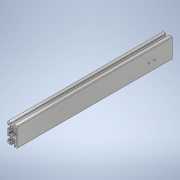
# Autodesk Inventor part: HFSF5-2040-320-TPW
Saved by Autodesk Inventor 2022 (Build 260153000, 153)
## iProperties
Category: PARTsolutions
Company: MISUMI
Created: 2022-12-05
Part Number: HFSF5-2040-320-TPW
Material: Generic
Catalog Web Link: www.cadenas.de
Description: NFS5-2040, NFSB5-2040, HFS5-2040, HFSB5-2040, CAF5-2040, NFSF5-2040, HFSF5-2040, HFSY5-2040-Aluminum Frames -5 Series-2Row Groove 20x40 mm Square -Specified Length
Vendor: MISUMI
Document SubType Name: Modeling
Designer: psAdmin
Manufacturer: MISUMI
Mass: 109.926 g
Surface Area: 1036.55 cm^2
Volume: 109.926 cm^3
Density: 1 g/cm^3
Appearance: アルミニウム - つや出し
PSOL_IDENT_0: {$CADENAS_DATA/23d-libs/misumi/metric/38_al_extrusions_blackets/5/hfs5_2040.prj},636 {VTYP=3D},{NB=H
PSOL_IDENT_1: FSF5-2040-320-TPW},{LINA=HFSF5-2040-320-TPW},{NN=NFS5-2040, NFSB5-2040, HFS5-2040, HFSB5-2040, CAF5-
PSOL_IDENT_2: 2040, NFSF5-2040, HFSF5-2040, HFSY5-2040},{DATE=30.11.2021 06:05:55},{GEOMDATE=23.09.2021 02:57:03},
PSOL_IDENT_3: {VERSION=},{LINEID=30},{WBVAR=L,ALT1,ALT2,ALT4,ALT5,CP5,DL5,DR5,ALT6,ALT9,ALT10,ALT11,HP6,NHL6,DL6,N
PSOL_IDENT_4: HR6,DR6,ALT7,ALT8,NH9,AH,BH,CH,DH,EH,NH10,AV,BV,CV,DV,EV,NH11,AP,BP,CP,DP,EP,ALT12,ALT13,Z,NH12,XA,X
PSOL_IDENT_5: B,XC,XD,XE,NH13,YA,YB,YC,YD,YE,ALT16,HP16,DL16,DR16,ALT17,HQ17,JLP,ALT18,HQ18,KLP,ALT20},{WBNUMERIC=
PSOL_IDENT_6: L,NH9,AH,BH,CH,DH,EH,NH10,AV,BV,CV,DV,EV,NH11,AP,BP,CP,DP,EP,NH12,XA,XB,XC,XD,XE,NH13,YA,YB,YC,YD,YE
PSOL_IDENT_7: ,HQ17,JLP,HQ18,KLP}  {NB=HFSF5-2040-320-TPW},{LINA=HFSF5-2040-320-TPW},{KT=DUMMY},{PN=HFSF5-2040-320
PSOL_IDENT_8: -TPW},{TPS=HFSF5-2040},{MAT=A6N01SS-T5 Aluminum Alloy},{ST=Clear Anodize},{FRMW=20},{FRMH=40},{FRD=4
PSOL_IDENT_9: .2},{L=320},{MASS=0.93},{SA=344},{LX=1.52x10^4},{LY=5.40x10^4},{ALT1=TPW},{M1=5},{DPL1=15},{DPR1=15}
PSOL_IDENT_10: ,{ALT1PN=-TPW},{ALT2=},{ALT2ALG= '','Not applicable' },{M2=0},{DP2=0},{ALT2PN=},{ALT4=},{ALT4ALG= ''
PSOL_IDENT_11: , 'w/o SC (High Precision Cut)', 'SC', 'with SC (High Precision Cut)' },{ALT4PN=},{ALT5=},{ALT5ALG= ''
PSOL_IDENT_12: ,'w/o 45 Degree Cut','1','with 45 Degree Cut' },{CP5=},{CP5ALG= '','N/A' },{DL5=},{DL5ALG= '','N/A'
PSOL_IDENT_13: },{DR5=},{DR5ALG= '','N/A' },{FRMLALT5=0},{FRMRALT5=0},{ALT5PN=},{ALT6=},{ALT6ALG= '','w/o Fastening
PSOL_IDENT_14: Location Wrench Access Hole Alterations','1','with Fastening Location Wrench Access Hole Alteration
PSOL_IDENT_15: s' },{ALT9=},{ALT9ALG= '','w/o Location Specified Wrench Access Hole Alteratons (Horizontal)','1','w
PSOL_IDENT_16: ith Location Specified Wrench Access Hole Alteratons (Horizontal)' },{ALT10=},{ALT10ALG= '','w/o Loc
PSOL_IDENT_17: ation Specified Wrench Access Hole Alteratons (Vertical)','1','with Location Specified Wrench Access
PSOL_IDENT_18: Hole Alteratons (Vertical)' },{ALT11=},{ALT11ALG= '','w/o Location Specified Wrench Access Hole Alt
PSOL_IDENT_19: eratons (Crisscross)','1','with Location Specified Wrench Access Hole Alteratons (Crisscross)' },{HP
PSOL_IDENT_20: 6=},{HP6ALG= '','N/A' },{NHL6=},{NHL6ALG= '','N/A' },{DL6=},{DL6ALG= '','N/A' },{NHR6=},{NHR6ALG= ''
PSOL_IDENT_21: ,'N/A' },{DR6=},{DR6ALG= '','N/A' },{HL6=0},{HL6D=0},{HR6=0},{HR6D=0},{J6=0},{J6D=0},{K6=0},{K6D=0},
PSOL_IDENT_22: {DD6=0.00},{DD6ALG=0},{ALT7=},{ALT7ALG= '','N/A' },{ALT8=},{ALT8ALG= '','N/A' },{ALT678PN=},{NH9=0},
PSOL_IDENT_23: {NH9MAX=5},{NH9ALG=[0]},{AH=0.0},{AHMIN=7},{AHMAX=315},{AHALG=[0]},{BH=0.0},{BHMIN=2},{BHMAX=317},{B
PSOL_IDENT_24: HALG=[0]},{CH=0.0},{CHMIN=2},{CHMAX=319},{CHALG=[0]},{DH=0.0},{DHMIN=2},{DHMAX=321},{DHALG=[0]},{EH=
PSOL_IDENT_25: 0.0},{EHMIN=2},{EHMAX=313},{EHALG=[0]},{NH10=0},{NH10MAX=5},{NH10ALG=[0]},{AV=0.0},{AVMIN=7},{AVMAX=
PSOL_IDENT_26: 315},{AVALG=[0]},{BV=0.0},{BVMIN=2},{BVMAX=317},{BVALG=[0]},{CV=0.0},{CVMIN=2},{CVMAX=319},{CVALG=[0
PSOL_IDENT_27: ]},{DV=0.0},{DVMIN=2},{DVMAX=321},{DVALG=[0]},{EV=0.0},{EVMIN=2},{EVMAX=313},{EVALG=[0]},{NH11=0},{N
PSOL_IDENT_28: H11MAX=5},{NH11ALG=[0]},{AP=0.0},{APMIN=7},{APMAX=315},{APALG=[0]},{BP=0.0},{BPMIN=2},{BPMAX=317},{B
PSOL_IDENT_29: PALG=[0]},{CP=0.0},{CPMIN=2},{CPMAX=319},{CPALG=[0]},{DP=0.0},{DPMIN=2},{DPMAX=321},{DPALG=[0]},{EP=
PSOL_IDENT_30: 0.0},{EPMIN=2},{EPMAX=313},{EPALG=[0]},{ALT9PN=},{ALT10PN=},{ALT11PN=},{ALT91011PN=},{ALT12=},{ALT12
PSOL_IDENT_31: ALG= '','w/o Counterbore Hole in Specified Position (Vertical)','1','with Counterbore Hole in Specif
PSOL_IDENT_32: ied Position (Vertical)' },{ALT13=},{ALT13ALG= '','N/A' },{Z=},{ZALG= '','N/A' },{DD12=0.0},{DD112=0
PSOL_IDENT_33: .0},{NH12=0},{NH12MAX=5},{NH12ALG=[0]},{XA=0.0},{XAMIN=7},{XAMAX=315},{XAALG=[0]},{XB=0.0},{XBMIN=2}
PSOL_IDENT_34: ,{XBMAX=317},{XBALG=[0]},{XC=0.0},{XCMIN=2},{XCMAX=319},{XCALG=[0]},{XD=0.0},{XDMIN=2},{XDMAX=321},{
PSOL_IDENT_35: XDALG=[0]},{XE=0.0},{XEMIN=2},{XEMAX=313},{XEALG=[0]},{NH13=0},{NH13MAX=5},{NH13ALG=[0]},{YA=0.0},{Y
PSOL_IDENT_36: AMIN=7},{YAMAX=315},{YAALG=[0]},{YB=0.0},{YBMIN=2},{YBMAX=317},{YBALG=[0]},{YC=0.0},{YCMIN=2},{YCMAX=
PSOL_IDENT_37: 319},{YCALG=[0]},{YD=0.0},{YDMIN=2},{YDMAX=321},{YDALG=[0]},{YE=0.0},{YEMIN=2},{YEMAX=313},{YEALG=[0
PSOL_IDENT_38: ]},{ALT12PN=},{ALT13PN=},{ALT1213PN=},{ALT16=},{ALT16ALG= '','w/o M Type Hole Alteration','1','with
PSOL_IDENT_39: M Type Hole Alteration' },{HP16=},{HP16ALG= '','N/A' },{DL16=},{DL16ALG= '','N/A' },{DR16=},{DR16ALG=
PSOL_IDENT_40: '','N/A' },{H116=0},{D16=0.0},{ALT16PN=},{ALT17=},{ALT17ALG= '','w/o L Type Hole Alteration (Top)','
PSOL_IDENT_41: 1','with L Type Hole Alteration (Top)' },{HQ17=0},{HQ17ALG=0},{JLP=0},{JLPMIN=4.9},{JLPMAX=0},{JLPAL
PSOL_IDENT_42: G=[0]},{L17=0},{D17=0.0},{ALT18=},{ALT18ALG= '','w/o L Type Hole Alteration (Bottom)','1','with L Ty
PSOL_IDENT_43: pe Hole Alteration (Bottom)' },{HQ18=0},{HQ18ALG=0},{KLP=0},{KLPMIN=4.9},{KLPMAX=0},{KLPALG=[0]},{L1
PSOL_IDENT_44: 8=0},{D18=0.0},{ALT1718PN=},{ALT20=},{ALT20PN=},{ERRORALT01=OK},{ERRORALT02=OK},{ERRORALT05=OK},{ERR
PSOL_IDENT_45: ORALT06091=OK},{ERRORALT06092=OK},{ERRORALT06093=OK},{ERRORALT06094=OK},{ERRORALT06101=OK},{ERRORALT
PSOL_IDENT_46: 06102=OK},{ERRORALT06103=OK},{ERRORALT06104=OK},{ERRORALT06111=OK},{ERRORALT06112=OK},{ERRORALT06113=
PSOL_IDENT_47: OK},{ERRORALT06114=OK},{ERRORALT06121=OK},{ERRORALT06122=OK},{ERRORALT06123=OK},{ERRORALT06124=OK},{
PSOL_IDENT_48: ERRORALT06131=OK},{ERRORALT06132=OK},{ERRORALT06133=OK},{ERRORALT06134=OK},{ERRORALT0616=OK},{ERRORA
PSOL_IDENT_49: LT06171=OK},{ERRORALT06172=OK},{ERRORALT06173=OK},{ERRORALT06181=OK},{ERRORALT06182=OK},{ERRORALT061
PSOL_IDENT_50: 83=OK},{ERRORALT0911=OK},{ERRORALT0913=OK},{ERRORALT0916=OK},{ERRORALT0917=OK},{ERRORALT0918=OK},{ER
PSOL_IDENT_51: RORALT1011=OK},{ERRORALT1012=OK},{ERRORALT1016=OK},{ERRORALT1017=OK},{ERRORALT1018=OK},{ERRORALT1112=
PSOL_IDENT_52: OK},{ERRORALT1113=OK},{ERRORALT1116=OK},{ERRORALT1117=OK},{ERRORALT1118=OK},{ERRORALT1216=OK},{ERROR
PSOL_IDENT_53: ALT1217=OK},{ERRORALT1218=OK},{ERRORALT1316=OK},{ERRORALT1317=OK},{ERRORALT1318=OK},{ERRORALT1617=OK
PSOL_IDENT_54: },{ERRORALT1618=OK},{ERRORPN=},{TFW=2},{COLOR=}
NB: HFSF5-2040-320-TPW
NN: NFS5-2040, NFSB5-2040, HFS5-2040, HFSB5-2040, CAF5-2040, NFSF5-2040, HFSF5-2040, HFSY5-2040
NT: Aluminum Frames -5 Series-2Row Groove 20x40 mm Square -Specified Length
NBSYN: $PN.
LINA: HFSF5-2040-320-TPW
CATALOG: Misumi
PN: HFSF5-2040-320-TPW
TPS: HFSF5-2040
MAT: A6N01SS-T5 Aluminum Alloy
ST: Clear Anodize
L: 320
MASS: 0.93
SA: 344
LX: 1.52x10^4
LY: 5.40x10^4
ALT1: with TPW (Tapping on Both Ends)
M1: 5
DPL1: 15
DPR1: 15
ALT2: Not applicable
M2: 0
DP2: 0
ALT4: w/o SC (High Precision Cut)
ALT5: w/o 45 Degree Cut
CP5: N/A
DL5: N/A
DR5: N/A
ALT6: w/o Fastening Location Wrench Access Hole Alterations
ALT9: w/o Location Specified Wrench Access Hole Alteratons (Horizontal)
ALT10: w/o Location Specified Wrench Access Hole Alteratons (Vertical)
ALT11: w/o Location Specified Wrench Access Hole Alteratons (Crisscross)
HP6: N/A
NHL6: N/A
DL6: N/A
NHR6: N/A
DR6: N/A
HL6D: 0
HR6D: 0
J6D: 0
K6D: 0
DD6: 0
ALT7: N/A
ALT8: N/A
NH9: 0
AH: 0
BH: 0
CH: 0
DH: 0
EH: 0
NH10: 0
AV: 0
BV: 0
CV: 0
DV: 0
EV: 0
NH11: 0
AP: 0
BP: 0
CP: 0
DP: 0
EP: 0
ALT12: w/o Counterbore Hole in Specified Position (Vertical)
ALT13: N/A
Z: N/A
DD12: 0
DD112: 0
NH12: 0
XA: 0
XB: 0
XC: 0
XD: 0
XE: 0
NH13: 0
YA: 0
YB: 0
YC: 0
YD: 0
YE: 0
ALT16: w/o M Type Hole Alteration
HP16: N/A
DL16: N/A
DR16: N/A
H116: 0
D16: 0
ALT17: w/o L Type Hole Alteration (Top)
HQ17: 0
JLP: 0
D17: 0
ALT18: w/o L Type Hole Alteration (Bottom)
HQ18: 0
KLP: 0
D18: 0
ALT20: w/o CW (End Face C Chamfering)
SUPPLIER: MISUMI
ARTICLENO: HFSF5-2040-320-TPW
BOMINFO: HFSF5-2040-320-TPW
CREATOR: CADENAS GmbH
Title: HFSF5-2040-320-TPW
Author: Cadenas PARTsolutions
Comments: Aluminum Frames -5 Series-2Row Groove 20x40 mm Square -Specified Length
Autodesk Inventor part; units mm, degrees
ref_plane "YZ Plane" through (0, 0, 0) normal (1, 0, 0) x (0, 1, 0)
ref_plane "XZ Plane" through (0, 0, 0) normal (0, 1, 0) x (-1, 0, 0)
ref_plane "XY Plane" through (0, 0, 0) normal (0, 0, 1) x (1, 0, 0)
sketch "Sketch_63" plane through (0, 0, 0) normal (0, 0, 1) x (1, 0, 0)
  line L0 (-10, -7) -> (-8, -7)
  line L1 (-8, -7) -> (-8, -4)
  line L2 (-8, -4) -> (-7.0607, -4)
  line L3 (-7.0607, -4) -> (-4, -7.0607)
  line L4 (-4, -7.0607) -> (-4, -9.4804)
  line L5 (-4, -9.4804) -> (-3.7, -10)
  line L6 (-3.7, -10) -> (-4, -10.5196)
  line L7 (-4, -10.5196) -> (-4, -12.9393)
  line L8 (-4, -12.9393) -> (-7.0607, -16)
  line L9 (-7.0607, -16) -> (-8, -16)
  line L10 (-8, -16) -> (-8, -13)
  line L11 (-8, -13) -> (-10, -13)
  line L12 (-10, -13) -> (-10, -19)
  arc A0 (-10, -19) -> (-9, -20) centre (-9, -19) ccw
  line L13 (-9, -20) -> (-3, -20)
  line L14 (-3, -20) -> (-3, -18)
  line L15 (-3, -18) -> (-6, -18)
  line L16 (-6, -18) -> (-6, -17.0607)
  line L17 (-6, -17.0607) -> (-2.9393, -14)
  line L18 (-2.9393, -14) -> (-0.5196, -14)
  line L19 (-0.5196, -14) -> (0, -13.7)
  line L20 (0, -13.7) -> (0.5196, -14)
  line L21 (0.5196, -14) -> (2.9393, -14)
  line L22 (2.9393, -14) -> (6, -17.0607)
  line L23 (6, -17.0607) -> (6, -18)
  line L24 (6, -18) -> (3, -18)
  line L25 (3, -18) -> (3, -20)
  line L26 (3, -20) -> (9, -20)
  arc A1 (9, -20) -> (10, -19) centre (9, -19) ccw
  line L27 (10, -19) -> (10, 19)
  arc A2 (10, 19) -> (9, 20) centre (9, 19) ccw
  line L28 (9, 20) -> (3, 20)
  line L29 (3, 20) -> (3, 18)
  line L30 (3, 18) -> (6, 18)
  line L31 (6, 18) -> (6, 17.0607)
  line L32 (6, 17.0607) -> (2.9393, 14)
  line L33 (2.9393, 14) -> (0.5196, 14)
  line L34 (0.5196, 14) -> (0, 13.7)
  line L35 (0, 13.7) -> (-0.5196, 14)
  line L36 (-0.5196, 14) -> (-2.9393, 14)
  line L37 (-2.9393, 14) -> (-6, 17.0607)
  line L38 (-6, 17.0607) -> (-6, 18)
  line L39 (-6, 18) -> (-3, 18)
  line L40 (-3, 18) -> (-3, 20)
  line L41 (-3, 20) -> (-9, 20)
  arc A3 (-9, 20) -> (-10, 19) centre (-9, 19) ccw
  line L42 (-10, 19) -> (-10, 13)
  line L43 (-10, 13) -> (-8, 13)
  line L44 (-8, 13) -> (-8, 16)
  line L45 (-8, 16) -> (-7.0607, 16)
  line L46 (-7.0607, 16) -> (-4, 12.9393)
  line L47 (-4, 12.9393) -> (-4, 10.5196)
  line L48 (-4, 10.5196) -> (-3.7, 10)
  line L49 (-3.7, 10) -> (-4, 9.4804)
  line L50 (-4, 9.4804) -> (-4, 7.0607)
  line L51 (-4, 7.0607) -> (-7.0607, 4)
  line L52 (-7.0607, 4) -> (-8, 4)
  line L53 (-8, 4) -> (-8, 7)
  line L54 (-8, 7) -> (-10, 7)
  line L55 (-10, 7) -> (-10, -7)
  line L56 (4, 12.9393) -> (4, 8.5)
  arc A4 (4, 8.5) -> (5, 7.5) centre (5, 8.5) ccw
  line L57 (5, 7.5) -> (7, 7.5)
  arc A5 (7, 7.5) -> (8, 8.5) centre (7, 8.5) ccw
  line L58 (8, 8.5) -> (8, 16)
  line L59 (8, 16) -> (7.0607, 16)
  line L60 (7.0607, 16) -> (4, 12.9393)
  line L61 (4, -12.9393) -> (7.0607, -16)
  line L62 (7.0607, -16) -> (8, -16)
  line L63 (8, -16) -> (8, -8.5)
  arc A6 (8, -8.5) -> (7, -7.5) centre (7, -8.5) ccw
  line L64 (7, -7.5) -> (5, -7.5)
  arc A7 (5, -7.5) -> (4, -8.5) centre (5, -8.5) ccw
  line L65 (4, -8.5) -> (4, -12.9393)
  line L66 (-8, 1.7) -> (-8, -1.7)
  arc A8 (-8, -1.7) -> (-7.7, -2) centre (-7.7, -1.7) ccw
  line L67 (-7.7, -2) -> (-7.0636, -2)
  arc A9 (-6.8515, -2.0879) -> (-7.0636, -2) centre (-7.0636, -2.3) ccw
  line L68 (-6.8515, -2.0879) -> (-2.9393, -6)
  line L69 (-2.9393, -6) -> (7, -6)
  arc A10 (7, -6) -> (8, -5) centre (7, -5) ccw
  line L70 (8, -5) -> (8, 5)
  arc A11 (8, 5) -> (7, 6) centre (7, 5) ccw
  line L71 (7, 6) -> (-2.9393, 6)
  line L72 (-2.9393, 6) -> (-6.8515, 2.0879)
  arc A12 (-7.0636, 2) -> (-6.8515, 2.0879) centre (-7.0636, 2.3) ccw
  line L73 (-7.0636, 2) -> (-7.7, 2)
  arc A13 (-7.7, 2) -> (-8, 1.7) centre (-7.7, 1.7) ccw
  constraints: 148 end point, 28 point on circle, 14 centre point
extrude "Extrusion1" add sketch "Sketch_63" against normal blind 320
sketch "Sketch2" plane through (0, 0, 0) normal (0, 0, 1) x (1, 0, 0)
  point P0 (0, 10)
hole "Hole1" at (0, 10, 0) direction (0, 0, -1) diameter 4.134 depth 15 countersink diameter 5 countersink angle 90 thread size "M5x0.8" class "6H" standard "ISO Metric profile"
pattern_linear "Rectangular Pattern1" count 2 spacing 20 along (0, -1, 0) of "Hole1"
sketch "Sketch3" plane through (0, 0, -320) normal (0, 0, -1) x (-1, 0, 0)
  point P0 (0, 10)
hole "Hole2" at (0, 10, -320) direction (0, 0, 1) diameter 4.134 depth 15 countersink diameter 5 countersink angle 90 thread size "M5x0.8" class "6H" standard "ISO Metric profile"
pattern_linear "Rectangular Pattern2" count 2 spacing 20 along (0, -1, 0) of "Hole2"
sketch "Sketch4" plane through (0, 10, -305) normal (0, 0, -1) x (-1, 0, 0)
  point P0 (0, 0)
hole "Hole3" at (0, 10, -305) direction (0, 0, 1) diameter 4.2 depth 290
pattern_linear "Rectangular Pattern3" count 2 spacing 20 along (0, -1, 0) of "Hole3"
ref_plane "C1_XY" through (0, 0, 0) normal (0, 0, 1) x (1, 0, 0)
ref_plane "C1_YZ" through (0, 0, 0) normal (1, 0, 0) x (0, 1, 0)
ref_plane "C1_ZX" through (0, 0, 0) normal (0, 1, 0) x (0, 0, 1)
sketch "スケッチ7" plane through (10, -19, 0) normal (1, 0, 0) x (0, 0, -1)
  line L0 (0, 0) -> (320, 0) projected
  line L1 (320, 38) -> (320, 0) projected
  point P0 (0, 19)
  point P1 (271.5, 16)
  point P2 (283.5, 16)
  dimension "d52" = 16
  dimension "d53" = 48.5
  dimension "d54" = 36.5
  measures "d52" distance from line of L0 point (271.5, 16)
  measures "d53" distance from line of L1 point (271.5, 16)
  measures "d54" distance from line of L1 point (283.5, 16)
hole "穴5" at (10, -3, -271.5) at (10, -3, -283.5) direction (-1, 0, 0) diameter 2.459 end through all thread size "M3x0.5" class "6H" standard "ANSI Metric M Profile"
body "Solid1"
